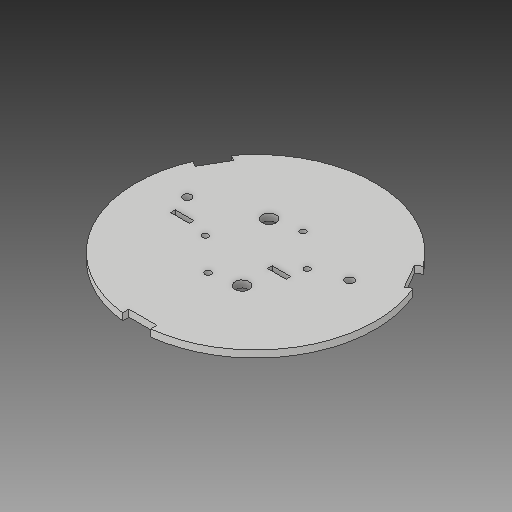
# Autodesk Inventor part: LUXCAN BASE DE MONTAJE LENTE
Saved by Autodesk Inventor 2018 (Build 220112000, 112)
## iProperties
Created: 2018-08-10
Part Number: LUXCAN BASE DE MONTAJE LENTE
Material: Generic
Document SubType Name: Sheet Metal
Designer: jocdurso
Density: 1 g/cm^3
Sheet Metal Rule: Default
Appearance: Default
Author: jocdurso
Autodesk Inventor part; units mm, degrees
ref_plane "YZ Plane" through (0, 0, 0) normal (1, 0, 0) x (0, 1, 0)
ref_plane "XZ Plane" through (0, 0, 0) normal (0, 1, 0) x (-1, 0, 0)
ref_plane "XY Plane" through (0, 0, 0) normal (0, 0, 1) x (1, 0, 0)
sketch "Sketch9" plane through (0, 3, 0) normal (0, 1, 0) x (1, 0, 0)
  line L0 (10.4056, -28.6) -> (-19.5944, -28.6)
  line L1 (-19.5944, -28.6) -> (-19.5944, -24.6)
  line L2 (-19.5944, -24.6) -> (10.4056, -24.6)
  line L3 (10.4056, -24.6) -> (10.4056, -28.6)
  point P0 (0, 0)
sketch "Sketch1" plane through (0, 0, 0) normal (0, 1, 0) x (-1, 0, 0)
  circle A0 centre (0, 0) radius 51.35
  dimension "d0" = 102.7
  measures "d0" diameter of A0
extrude "Plate1" add sketch "Sketch1" along normal blind 3
sketch "Sketch2" plane through (0, 0, 0) normal (0, 1, 0) x (-1, 0, 0)
  line L0 (6, 48.2983) -> (-6, 48.2983)
  line L1 (-6, 48.2983) -> (-6, 53.6983)
  line L2 (-6, 53.6983) -> (6, 53.6983)
  line L3 (6, 53.6983) -> (6, 48.2983)
  line L4 (6, 48.2983) -> (-6, 48.2983)
  line L5 (-6, 48.2983) -> (-6, 50.9983)
  line L6 (-6, 50.9983) -> (6, 50.9983)
  line L7 (6, 50.9983) -> (6, 48.2983)
  circle A0 centre (0, 0) radius 51.35 projected
  point P0 (0, 48.2983)
  point P1 (0, 48.2983)
  dimension "d2" = 2.7
  dimension "d3" = 12
  constraints: 16 end point, 4 midpoint, 4 parallel, 2 horizontal, 2 perpendicular, 1 vertical alignment, 2 other
  measures "d2" distance between parallel lines of L0 L6
  measures "d3" distance of L1.end L2.end
extrude "Cut1" cut sketch "Sketch2" along normal through all contours L0 L1 L6 L3 | A0 L1 L2 L3 | L6 A0
pattern_circular "Circular Pattern1" count 3 over 360 about axis through (0, -10, 0) along (0, 1, 0) of "Cut1"
sketch "Sketch3" plane through (0, 0, 0) normal (0, 1, 0) x (-1, 0, 0)
  point P0 (0, 0)
  point P1 (35.1, -5.8)
  point P2 (-30.6, -9.7)
  dimension "d9" = 5.8
  dimension "d10" = 35.1
  dimension "d11" = 9.7
  dimension "d12" = 30.6
  measures "d9" vertical distance of point (0, 0) point (35.1, -5.8)
  measures "d10" horizontal distance of point (0, 0) point (35.1, -5.8)
  measures "d11" vertical distance of point (0, 0) point (-30.6, -9.7)
  measures "d12" horizontal distance of point (0, 0) point (-30.6, -9.7)
hole "Hole1" at (-35.1, 0, -5.8) at (30.6, 0, -9.7) direction (0, 1, 0) diameter 3.6 end through all
sketch "Sketch4" plane through (0, 3, 0) normal (0, 1, 0) x (1, 0, 0)
  point P0 (0, 0)
  point P1 (-16.9, -4.7)
  point P2 (17.3, 4.8)
  dimension "d20" = 4.7
  dimension "d21" = 16.9
  dimension "d22" = 17.3
  dimension "d23" = 4.8
  measures "d20" vertical distance of point (0, 0) point (-16.9, -4.7)
  measures "d21" horizontal distance of point (0, 0) point (-16.9, -4.7)
  measures "d22" horizontal distance of point (17.3, 4.8) point (0, 0)
  measures "d23" vertical distance of point (0, 0) point (17.3, 4.8)
hole "Hole2" at (-16.9, 3, 4.7) at (17.3, 3, -4.8) direction (0, -1, 0) diameter 2.6 end through all
sketch "Sketch5" plane through (0, 3, 0) normal (0, 1, 0) x (1, 0, 0)
  point P0 (0, 0)
  point P1 (-9.5, 15.3)
  point P2 (9.5, -15.3)
  dimension "d31" = 9.5
  dimension "d32" = 15.3
  dimension "d33" = 9.5
  dimension "d34" = 15.3
  measures "d31" horizontal distance of point (0, 0) point (-9.5, 15.3)
  measures "d32" vertical distance of point (-9.5, 15.3) point (0, 0)
  measures "d33" horizontal distance of point (0, 0) point (9.5, -15.3)
  measures "d34" vertical distance of point (0, 0) point (9.5, -15.3)
hole "Hole3" at (-9.5, 3, -15.3) at (9.5, 3, 15.3) direction (0, -1, 0) diameter 6 end through all
sketch "Sketch6" plane through (0, 3, 0) normal (0, 1, 0) x (1, 0, 0)
  line L0 (-32.9, -1.5) -> (-24.9, -1.5)
  line L1 (-24.9, -1.5) -> (-24.9, -3.5)
  line L2 (-24.9, -3.5) -> (-32.9, -3.5)
  line L3 (-32.9, -3.5) -> (-32.9, -1.5)
  line L4 (8.6, -1.5) -> (16.6, -1.5)
  line L5 (16.6, -1.5) -> (16.6, -3.5)
  line L6 (16.6, -3.5) -> (8.6, -3.5)
  line L7 (8.6, -3.5) -> (8.6, -1.5)
  line L8 (-19.5944, -24.6) -> (10.4056, -24.6)
  line L9 (10.4056, -24.6) -> (10.4056, -28.6)
  line L10 (10.4056, -28.6) -> (-19.5944, -28.6)
  line L11 (-19.5944, -28.6) -> (-19.5944, -24.6)
  point P0 (0, 0)
  dimension "d42" = 8
  dimension "d43" = 8
  dimension "d44" = 33.5
  dimension "d45" = 24.9
  dimension "d46" = 2
  dimension "d47" = 1.5
  dimension "d48" = 21.1
  dimension "d49" = 30
  dimension "d50" = 4
  constraints: 24 end point, 6 parallel, 3 horizontal, 3 perpendicular, 2 point on line
  measures "d42" distance of L4.start L4.end
  measures "d43" distance of L0.start L0.end
  measures "d44" distance between parallel lines of L7 L1
  measures "d45" distance from line of L1 point (0, 0)
  measures "d46" distance of L2.end L0.start
  measures "d47" distance from line of L0 point (0, 0)
  measures "d48" distance between parallel lines of L8 L2
  measures "d49" distance of L9.end L10.end
  measures "d50" distance of L8.end L9.end
extrude "Cut2" cut sketch "Sketch6" against normal blind 3
sketch "Sketch7" plane through (0, 3, 0) normal (0, 1, 0) x (1, 0, 0)
  point P0 (0, 0)
  point P1 (0, 18)
  point P2 (0, -18)
  dimension "d53" = 18
  dimension "d54" = 18
  constraints: 2 vertical alignment
  measures "d53" distance of point (0, 0) point (0, 18)
  measures "d54" distance of point (0, 0) point (0, -18)
hole "Hole4" [suppressed]
sketch "Sketch8" plane through (0, 3, 0) normal (0, 1, 0) x (1, 0, 0)
  circle A0 centre (0, 0) radius 18
  point P0 (2.5, 17.8255)
  point P1 (-2.5, -17.8255)
  dimension "d62" = 36
  dimension "d63" = 2.5
  dimension "d64" = 2.5
  constraints: 2 point on circle, 1 centre point, 1 coincident
  measures "d62" diameter of A0
  measures "d63" horizontal distance of point (0, 0) A0.start
  measures "d64" horizontal distance of point (0, 0) A0.end
hole "Hole5" at (2.5, 3, -17.8255) at (-2.5, 3, 17.8255) direction (0, -1, 0) diameter 2.6 end through all
sheet face with bend "Face2" sketch "Sketch9" thickness 3 toward (0, -1, 0) bend radius 3
bend "Bend1"
equation "\"d4\" = Thickness"
equation "\"d18\" = Thickness"
equation "\"d29\" = Thickness"
equation "\"d40\" = Thickness"
equation "\"d51\" = Thickness"
equation "\"d60\" = Thickness"
equation "\"d70\" = Thickness"
equation "\"d77\" = Thickness"
equation "\"d72\" = BendRadius"
equation "\"d73\" = BendReliefWidth"
equation "\"d75\" = MinimumRemnant"
equation "\"d74\" = BendReliefDepth"
equation "\"d76\" = BendRadius"
equation "\"BendRadius\" = Thickness"
equation "\"BendReliefWidth\" = Thickness"
equation "\"BendReliefDepth\" = 0.5 * Thickness"
equation "\"CornerReliefSize\" = 4 * Thickness"
equation "\"MinimumRemnant\" = 2 * Thickness"
equation "\"TransitionRadius\" = BendRadius"
equation "\"JacobiRadiusSize\" = BendRadius"
equation "\"GapSize\" = Thickness"
equation "\"d1\" = BendRadius"
equation "\"Thickness\" = 3"
body "Solid1"
